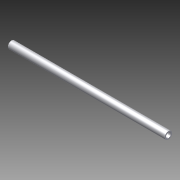
# Autodesk Inventor part: 252805
Saved by Autodesk Inventor 2011 (Build 150239000, 239)
## iProperties
Category: Miscellaneous
Company: Autodesk Inc.
Created: 2008-12-09
Part Number: 252805
Document SubType Name: Modeling
Designer: Autodesk Inc.
Density: 1.13 g/cm^3
Material: Nylon-6/6
Catalog Web Link: http://www.fastenersuperstore.com/index2.cfm
Description: Spacer
Vendor: Fastener Superstore
Mass: 1.1507 g
Surface Area: 25.4548 cm^2
Volume: 1.01832 cm^3
Author: Autodesk Inc.
Autodesk Inventor part; units mm, degrees
ref_plane "YZ Plane" through (0, 0, 0) normal (1, 0, 0) x (0, 1, 0)
ref_plane "XZ Plane" through (0, 0, 0) normal (0, 1, 0) x (-1, 0, 0)
ref_plane "XY Plane" through (0, 0, 0) normal (0, 0, 1) x (1, 0, 0)
sketch "Sketch1" plane through (0, 0, 0) normal (0, 0, 1) x (1, 0, 0)
  circle A0 centre (0, 0) radius 2.3813
  circle A1 centre (0, 0) radius 1.5748
  dimension "d0" = 4.7625
  dimension "d1" = 3.1496
  constraints: 2 centre point, 1 coincident
  measures "d0" diameter of A0
  measures "d1" diameter of A1
extrude "Extrusion1" add sketch "Sketch1" against normal blind 101.6
body "Solid1"
